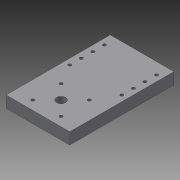
# Autodesk Inventor part: Lead_Screw_Fixture_Base
Saved by Autodesk Inventor 2015 (Build 190159000, 159)
## iProperties
Created: 2014-12-21
Part Number: Lead_Screw_Fixture_Base
Material: Generic
Document SubType Name: Modeling
Designer: Drew
Density: 1 g/cm^3
Appearance: Default
Author: Drew
Autodesk Inventor part; units mm, degrees
ref_plane "YZ Plane" through (0, 0, 0) normal (1, 0, 0) x (0, 1, 0)
ref_plane "XZ Plane" through (0, 0, 0) normal (0, 1, 0) x (-1, 0, 0)
ref_plane "XY Plane" through (0, 0, 0) normal (0, 0, 1) x (1, 0, 0)
sketch "Sketch1" plane through (0, 0, 0) normal (0, 1, 0) x (-1, 0, 0)
  line L0 (-34.925, -57.15) -> (34.925, -57.15)
  line L1 (34.925, -57.15) -> (34.925, 57.15)
  line L2 (34.925, 57.15) -> (-34.925, 57.15)
  line L3 (-34.925, 57.15) -> (-34.925, -57.15)
  line L4 (-34.925, -57.15) -> (34.925, 57.15) construction
  line L5 (34.925, -57.15) -> (-34.925, 57.15) construction
  point P0 (0, 0)
  dimension "d0" = 69.85
  dimension "d1" = 114.3
  constraints: 12 end point, 2 midpoint, 2 parallel, 1 horizontal, 1 perpendicular
  measures "d0" distance of L0.start L0.end
  measures "d1" distance of L0.end L1.end
extrude "Extrusion1" add sketch "Sketch1" along normal blind 12.7
sketch "Sketch2" plane through (0, 12.7, 0) normal (0, 1, 0) x (1, 0, 0)
  line L0 (0, 0) -> (0, -188.6697)
  line L1 (43.5518, -31.75) -> (-58.772, -31.75)
  line L2 (52.9625, 0) -> (-57.3554, 0)
  line L3 (-34.925, -57.15) -> (34.925, -57.15) projected
  point P0 (15.494, -47.25)
  point P1 (15.494, -16.25)
  point P2 (-15.494, -47.25)
  point P3 (-15.494, -16.25)
  point P4 (0, -31.75)
  dimension "d7" = 31
  dimension "d8" = 30.988
  dimension "d46" = 25.4
  constraints: 6 end point, 3 horizontal, 3 symmetric about line, 2 point on line, 1 perpendicular, 1 vertical
  measures "d7" diameter of point (15.494, -47.25) L1
  measures "d8" diameter of point (15.494, -47.25) L0
  measures "d46" distance between parallel lines of L1 L3
hole "Hole1" at (15.494, 12.7, 47.25) at (15.494, 12.7, 16.25) at (-15.494, 12.7, 16.25) at (-15.494, 12.7, 47.25) direction (0, -1, 0) diameter 3.5 end through all
sketch "Sketch4" plane through (0, 12.7, 0) normal (0, 1, 0) x (1, 0, 0)
  circle A0 centre (15.494, -16.25) radius 1.75 projected
  circle A1 centre (-15.494, -47.25) radius 1.75 projected
  line L0 (15.494, -16.25) -> (-15.494, -47.25)
  circle A2 centre (-15.494, -16.25) radius 1.75 projected
  circle A3 centre (15.494, -47.25) radius 1.75 projected
  line L1 (-15.494, -16.25) -> (15.494, -47.25)
  point P0 (0, 0)
  point P1 (0, -31.75)
  constraints: 4 end point, 1 midpoint
hole "Hole2" at (0, 12.7, 31.75) direction (0, -1, 0) diameter 10 end through all
sketch "Sketch6" plane through (0, 12.7, 0) normal (0, 1, 0) x (1, 0, 0)
  line L0 (0, -77.2056) -> (0, 91.7239)
  line L1 (-28.575, 6.35) -> (-28.575, 44.45)
  line L2 (-34.925, 57.15) -> (-34.925, -57.15) projected
  line L3 (-34.925, 0) -> (-34.925, 57.15)
  line L4 (28.575, 6.35) -> (28.575, 44.45)
  line L5 (-64.5272, 0) -> (76.1693, 0)
  line L6 (34.925, 57.15) -> (-34.925, 57.15)
  line L7 (34.925, 57.15) -> (-34.925, 57.15) projected
  point P0 (0, 0)
  point P1 (-28.575, 19.05)
  point P2 (-28.575, 31.75)
  point P3 (28.575, 19.05)
  point P4 (28.575, 31.75)
  dimension "d29" = 12.7
  dimension "d30" = 12.7
  dimension "d31" = 12.7
  dimension "d34" = 6.35
  dimension "d44" = 12.7
  constraints: 12 end point, 5 point on line, 4 symmetric about line, 3 vertical, 1 collinear, 1 horizontal, 1 midpoint
  measures "d29" distance of point (-28.575, 19.05) L1.start
  measures "d30" distance of point (-28.575, 31.75) point (-28.575, 19.05)
  measures "d31" distance of L1.end point (-28.575, 31.75)
  measures "d34" distance between parallel lines of L2 L1
  measures "d44" distance from line of L6 L4.end
hole "Hole3" at (-28.575, 12.7, -6.35) at (-28.575, 12.7, -19.05) at (-28.575, 12.7, -31.75) at (-28.575, 12.7, -44.45) at (28.575, 12.7, -44.45) at (28.575, 12.7, -31.75) at (28.575, 12.7, -19.05) at (28.575, 12.7, -6.35) direction (0, -1, 0) diameter 3.5 end through all
equation "\"d30\" = d29"
equation "\"d31\" = d30"
body "Solid1"
